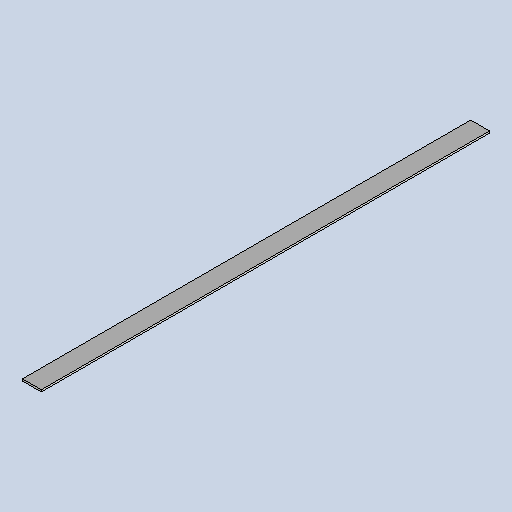
# Autodesk Inventor part: PNS waste water bin 08
Saved by Autodesk Inventor 2025.3 (Build 293356030, 356C)
## iProperties
Created: 2025-09-03
Part Number: PNS waste water bin 08
Material: Generic
Document SubType Name: Sheet Metal
Designer: admin
Density: 1 g/cm^3
Sheet Metal Rule: Default
Appearance: Default
Flat Pattern Width: 2 cm
Flat Pattern Length: 47.5 cm
Flat Pattern Area: 95 cm^2
Sheet Metal Width: 20,000 mm
Sheet Metal Length: 475,000 mm
Sheet Metal Area: 9500,000 mm^2
Mass: 19 g
Surface Area: 209.8 cm^2
Volume: 19 cm^3
Author: admin
Autodesk Inventor part; units mm, degrees
ref_plane "YZ Plane" through (0, 0, 0) normal (1, 0, 0) x (0, 1, 0)
ref_plane "XZ Plane" through (0, 0, 0) normal (0, 1, 0) x (-1, 0, 0)
ref_plane "XY Plane" through (0, 0, 0) normal (0, 0, 1) x (1, 0, 0)
sketch "Sketch1" plane through (0, 0, 0) normal (0, 0, 1) x (1, 0, 0)
  line L0 (10, 237.5) -> (-10, -237.5) construction
  line L1 (-10, -237.5) -> (10, -237.5)
  line L2 (10, -237.5) -> (10, 237.5)
  line L3 (10, 237.5) -> (-10, 237.5)
  line L4 (-10, 237.5) -> (-10, -237.5)
  line L5 (-10, -237.5) -> (10, 237.5) construction
  line L6 (10, -237.5) -> (-10, 237.5) construction
  point P0 (0, 0)
  point P1 (-180, -237.5)
  point P2 (-10, -192.5)
  dimension "d2" = 20
  dimension "d18" = 475
  measures "d2" distance of L3.end L2.end
  measures "d18" distance of L1.end L2.end
extrude "Plate1" add sketch "Sketch1" along normal blind 2
equation "\"d3\" = Thickness"
equation "\"BendRadius\" = Thickness"
equation "\"BendReliefWidth\" = Thickness"
equation "\"BendReliefDepth\" = 0.5 * Thickness"
equation "\"CornerReliefSize\" = 4 * Thickness"
equation "\"MinimumRemnant\" = 2 * Thickness"
equation "\"TransitionRadius\" = BendRadius"
equation "\"JacobiRadiusSize\" = BendRadius"
equation "\"GapSize\" = Thickness"
equation "\"Thickness\" = 2"
body "Solid1"
